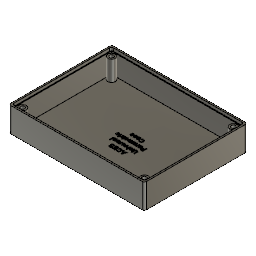
ACESUniversalParametricCase (Autodesk Fusion 360 design; units mm, degrees)
Autodesk Fusion 360 part; units mm, degrees
sketch "PCB" plane through (0, 0, 0) normal (0, 0, 1) x (1, 0, 0)
  line L0 (0, 0) -> (160, 0)
  line L1 (160, 0) -> (160, 120)
  line L2 (160, 120) -> (0, 120)
  line L3 (0, 120) -> (0, 0)
  line L4 (-0.5, -0.5) -> (160.5, -0.5)
  line L5 (160.5, -0.5) -> (160.5, 120.5)
  line L6 (160.5, 120.5) -> (-0.5, 120.5)
  line L7 (-0.5, 120.5) -> (-0.5, -0.5)
  line L8 (159.5, 0.5) -> (159.5, 119.5)
  line L9 (159.5, 119.5) -> (0.5, 119.5)
  line L10 (0.5, 119.5) -> (0.5, 0.5)
  line L11 (0.5, 0.5) -> (159.5, 0.5)
  line L12 (162.5, 122.5) -> (-2.5, 122.5)
  line L13 (-2.5, 122.5) -> (-2.5, -2.5)
  line L14 (-2.5, -2.5) -> (162.5, -2.5)
  line L15 (162.5, -2.5) -> (162.5, 122.5)
  dimension "d7" = 160
  dimension "d8" = 120
  dimension "d30" = 0.5
  dimension "d32" = 2.5
  constraint horizontal L0
  constraint vertical L1
  constraint horizontal L2
  constraint vertical L3
  constraint coincident L0.start L3.end
  measures "d7" distance of L0.start L0.end
  measures "d8" distance of L0.start L2.end
sketch "Piers" plane through (0, 0, 0) normal (0, 0, 1) x (1, 0, 0)
  line L0 (160, 120) -> (0, 120)
  circle A0 centre (6, 114) radius 4.5
  circle A1 centre (6, 114) radius 2.5
  line L1 (0, 120) -> (0, 0)
  line L2 (0, 0) -> (160, 0)
  circle A2 centre (6, 6) radius 4.5
  circle A3 centre (6, 6) radius 2.5
  line L3 (160, 0) -> (160, 120)
  circle A4 centre (154, 114) radius 4.5
  circle A5 centre (154, 114) radius 2.5
  circle A6 centre (154, 6) radius 4.5
  circle A7 centre (154, 6) radius 2.5
  point P0 (6, 114)
  point P1 (0, 120)
  point P2 (6, 6)
  point P3 (154, 114)
  point P4 (154, 6)
  point P5 (154, 6)
  dimension "d10" = 6
  dimension "d11" = 6
  dimension "d13" = 9
  dimension "d15" = 5
  dimension "d16" = 6
  dimension "d17" = 6
  dimension "d18" = 9
  dimension "d19" = 5
  dimension "d20" = 6
  dimension "d21" = 6
  dimension "d22" = 9
  dimension "d23" = 5
  dimension "d24" = 6
  dimension "d25" = 6
  dimension "d26" = 9
  dimension "d27" = 5
  constraint coincident P0 A0.centre
  constraint coincident P2 A2.centre
  constraint coincident P3 A4.centre
  constraint coincident P5 P4
  constraint concentric A6 A7
  measures "d10" horizontal distance of P0 L0.end
  measures "d11" distance of P0 L0
  measures "d13" diameter of A0
  measures "d15" diameter of A1
  measures "d16" distance of P2 L1
  measures "d17" distance of P2 L2
  measures "d18" diameter of A2
  measures "d19" diameter of A3
  measures "d20" distance of P3 L3
  measures "d21" distance of L0 P3
  measures "d22" diameter of A4
  measures "d23" diameter of A5
  measures "d24" distance of L3 P5
  measures "d25" distance of L2 P5
  measures "d26" diameter of A6
  measures "d27" diameter of A7
extrude "Extrude1" add sketch "Piers" along normal blind 26.4 contours A4 makes body 1
extrude "Extrude2" add sketch "Piers" along normal blind 21 contours A5 bodies 1
extrude "Extrude3" add sketch "Piers" along normal blind 21 separate body contours A7 makes body 2
extrude "Extrude4" add sketch "Piers" along normal blind 26.4 contours A6 bodies 2
extrude "Extrude5" add sketch "Piers" along normal blind 21 separate body contours A3 makes body 3
extrude "Extrude6" add sketch "Piers" along normal blind 26.4 contours A2 bodies 3
extrude "Extrude7" add sketch "Piers" along normal blind 21 separate body contours A1 makes body 4
extrude "Extrude8" add sketch "Piers" along normal blind 26.4 contours A0 bodies 4
extrude "Extrude9" cut sketch "PCB" along normal blind 2 contours L8 L9 L10 L11 bodies 1 2 3 4
extrude "Extrude10" add sketch "PCB" along normal blind 2 contours L8 L9 L10 L11 bodies 1 2 3 4
extrude "Extrude11" add sketch "PCB" along normal blind 26.4 contours L0 L1 L2 L3 bodies 1
extrude "Extrude12" add sketch "PCB" along normal blind 26.4 contours L4 L5 L6 L7 bodies 1
extrude "Extrude13" add sketch "PCB" along normal blind 30 contours L12 L13 L14 L15 bodies 1
fillet "Fillet1" radius 2.54 4 edges at (162.5, -2.5, 15) (-2.5, -2.5, 15) (162.5, 122.5, 15) (-2.5, 122.5, 15) on bodies 1
fillet "Fillet2" radius 2.54 1 edges at (160.5, -0.5, 28.2) on bodies 1
fillet "Fillet3" radius 2.54 1 edges at (-0.5, 120.5, 28.2) on bodies 1
fillet "Fillet4" radius 2.54 1 edges at (-0.5, -0.5, 28.2) on bodies 1
fillet "Fillet5" radius 2.54 1 edges at (160.5, 120.5, 28.2) on bodies 1
sketch "Text" plane through (0, 0, 2) normal (0, 0, 1) x (-1, 0, 0)
  circle A0 centre (-6, -6) radius 4.5
  circle A1 centre (-154, -114) radius 4.5
  circle A2 centre (-154, -6) radius 4.5
  circle A3 centre (-6, -114) radius 4.5
  line L0 (-0.5, -0.5) -> (-159.5, -0.5)
  line L1 (-159.5, -0.5) -> (-159.5, -119.5)
  line L2 (-159.5, -119.5) -> (-0.5, -119.5)
  line L3 (-0.5, -119.5) -> (-0.5, -0.5)
  line L4 (-124.729, -92.8924) -> (-40.8435, -92.8924) construction
  line L5 (-40.8435, -92.8924) -> (-40.8435, -19.5007) construction
  line L6 (-40.8435, -19.5007) -> (-124.729, -19.5007) construction
  line L7 (-124.729, -19.5007) -> (-124.729, -92.8924) construction
  dimension "d80" = 5
  text T0 "ACES\nUniversal\nParametric\nCase" font "Arial" height 5 bold align centre middle in box 83.8855 x 73.3917 at (-124.729, -92.8924) x (1, 0) y (0, 1) spacing 1
extrude "Extrude15" cut sketch "Text" against normal blind 1.5 text T0 bodies 1
equation "pcbWidth = 160 mm"
equation "pcbHeight = 120 mm"
equation "d7 = pcbWidth"
equation "d8 = pcbHeight"
equation "pierCornerOffset = 6 mm"
equation "d10 = pierCornerOffset"
equation "d11 = pierCornerOffset"
equation "pierOuterDiameter = 9 mm"
equation "d13 = pierOuterDiameter"
equation "pierInnerDiameter = 5 mm"
equation "d15 = pierInnerDiameter"
equation "d16 = pierCornerOffset"
equation "d17 = pierCornerOffset"
equation "d18 = pierOuterDiameter"
equation "d19 = pierInnerDiameter"
equation "d20 = pierCornerOffset"
equation "d21 = pierCornerOffset"
equation "d22 = pierOuterDiameter"
equation "d23 = pierInnerDiameter"
equation "d24 = pierCornerOffset"
equation "d25 = pierCornerOffset"
equation "d26 = pierOuterDiameter"
equation "d27 = pierInnerDiameter"
equation "pcbOffset = 0.5 mm"
equation "wallThickness = 2 mm"
equation "d30 = pcbOffset"
equation "d31 = -pcbOffset"
equation "d32 = pcbOffset + wallThickness"
equation "pierDepth = 7 mm"
equation "pcbThickness = 1.6 mm"
equation "caseHeight = 30 mm"
equation "pierHeight = caseHeight - pcbThickness - wallThickness"
equation "pierBaseHeight = caseHeight - pierDepth - wallThickness"
equation "d38 = pierHeight"
equation "d40 = pierBaseHeight"
equation "d42 = pierBaseHeight"
equation "d44 = pierHeight"
equation "d46 = pierBaseHeight"
equation "d48 = pierHeight"
equation "d50 = pierBaseHeight"
equation "d52 = pierHeight"
equation "d54 = wallThickness"
equation "d56 = wallThickness"
equation "d58 = pierHeight"
equation "d60 = pierHeight"
equation "d62 = caseHeight"
equation "filletRadius = 2.54 mm"
equation "d66 = filletRadius"
equation "d68 = filletRadius"
equation "d70 = filletRadius"
equation "d72 = filletRadius"
equation "d74 = filletRadius"
equation "textThickness = 1.5 mm"
equation "d82 = -textThickness"
